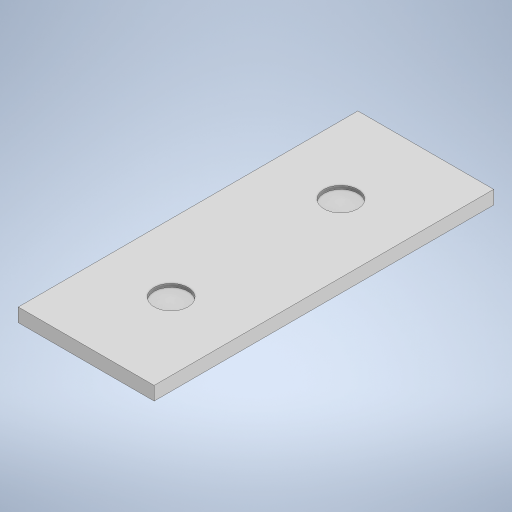
# Autodesk Inventor part: PortaHerramienta2
Saved by Autodesk Inventor 2024 (Build 280153000, 153)
## iProperties
Created: 2023-11-06
Part Number: PortaHerramienta2
Material: Generic
Document SubType Name: Modeling
Designer: Juan_Daleman
Density: 1 g/cm^3
Appearance: Default
Author: Juan_Daleman
Autodesk Inventor part; units mm, degrees
ref_plane "YZ Plane" through (0, 0, 0) normal (1, 0, 0) x (0, 1, 0)
ref_plane "XZ Plane" through (0, 0, 0) normal (0, 1, 0) x (-1, 0, 0)
ref_plane "XY Plane" through (0, 0, 0) normal (0, 0, 1) x (1, 0, 0)
sketch "Sketch1" plane through (0, 0, 0) normal (0, 1, 0) x (-1, 0, 0)
  line L0 (0, 0) -> (20, 0)
  line L1 (20, 0) -> (20, -50)
  line L2 (20, -50) -> (0, -50)
  line L3 (0, -50) -> (0, 0)
  dimension "d0" = 20
  dimension "d1" = 50
  constraints: 8 end point, 2 parallel, 1 horizontal, 1 perpendicular
  measures "d0" distance of L1.end L2.end
  measures "d1" distance of L0.end L1.end
extrude "Extrusion1" add sketch "Sketch1" along normal blind 2
sketch "Sketch2" plane through (0, 2, 0) normal (0, 1, 0) x (1, 0, 0)
  line L0 (-20, 0) -> (0, 0) projected
  line L1 (-10, 0) -> (-10, 50) construction
  line L2 (0, 50) -> (-20, 50) projected
  line L3 (-10, 0) -> (-10, 25) construction
  line L4 (-10, 25) -> (-10, 50) construction
  circle A0 centre (-10, 12.5) radius 2.5
  circle A1 centre (-10, 37.5) radius 2.5
  dimension "d4" = 5
  dimension "d5" = 5
  constraints: 6 end point, 5 midpoint, 2 centre point, 1 collinear
  measures "d4" diameter of A0
  measures "d5" diameter of A1
extrude "Extrusion2" cut sketch "Sketch2" against normal blind 0.5
body "Solid1"
